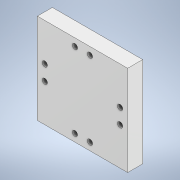
# Autodesk Inventor part: 土台
Saved by Autodesk Inventor 2021 (Build 250183000, 183)
## iProperties
Created: 2021-10-07
Part Number: 土台
Material: 一般
Document SubType Name: Modeling
Designer: ryusei
Density: 1 g/cm^3
Appearance: 滑らか - 白
Author: ryusei
Autodesk Inventor part; units mm, degrees
ref_plane "YZ Plane" through (0, 0, 0) normal (1, 0, 0) x (0, 1, 0)
ref_plane "XZ Plane" through (0, 0, 0) normal (0, 1, 0) x (-1, 0, 0)
ref_plane "XY Plane" through (0, 0, 0) normal (0, 0, 1) x (1, 0, 0)
sketch "スケッチ1" plane through (0, 0, 0) normal (0, 0, 1) x (1, 0, 0)
  line L0 (0, 0) -> (60, 0)
  line L1 (60, 0) -> (60, 60)
  line L2 (60, 60) -> (0, 60)
  line L3 (0, 60) -> (0, 0)
  dimension "d0" = 60
  dimension "d1" = 60
  constraints: 8 end point, 2 parallel, 1 horizontal, 1 perpendicular
  measures "d0" distance between parallel lines of L1 L3
  measures "d1" distance between parallel lines of L0 L2
extrude "押し出し1" add sketch "スケッチ1" along normal blind 10
sketch "スケッチ2" plane through (0, 0, 10) normal (0, 0, 1) x (1, 0, 0)
  line L0 (60, 60) -> (0, 60) projected
  line L1 (60, 0) -> (60, 60) projected
  line L2 (0, 0) -> (60, 0) projected
  line L3 (30, 60) -> (30, 0)
  point P0 (35, 55)
  point P1 (55, 35)
  point P2 (55, 25)
  point P3 (35, 5)
  point P4 (25, 55)
  point P5 (5, 35)
  point P6 (5, 25)
  point P7 (25, 5)
  dimension "d4" = 5
  dimension "d5" = 5
  dimension "d6" = 5
  dimension "d7" = 5
  dimension "d8" = 25
  dimension "d9" = 25
  dimension "d10" = 25
  dimension "d11" = 25
  constraints: 4 symmetric about line, 2 end point, 2 midpoint
  measures "d4" distance from line of L0 point (35, 55)
  measures "d5" distance from line of L1 point (55, 35)
  measures "d6" distance from line of L1 point (55, 25)
  measures "d7" distance from line of L2 point (35, 5)
  measures "d8" distance from line of L2 point (55, 25)
  measures "d9" distance from line of L1 point (35, 5)
  measures "d10" distance from line of L0 point (55, 35)
  measures "d11" distance from line of point (35, 55) L1
hole "穴1" at (35, 55, 10) at (55, 35, 10) at (55, 25, 10) at (35, 5, 10) at (25, 55, 10) at (5, 35, 10) at (5, 25, 10) at (25, 5, 10) direction (0, 0, -1) diameter 3.5 end through all
